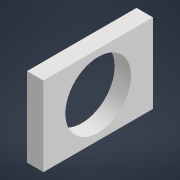
# Autodesk Inventor part: Part1
Saved by Autodesk Inventor 2022 (Build 260153000, 153)
## iProperties
Created: 2021-11-03
Part Number: Part1
Material: Generic
Document SubType Name: Modeling
Designer: 17185
Density: 1 g/cm^3
Appearance: Default
Author: 17185
Autodesk Inventor part; units mm, degrees
ref_plane "YZ Plane" through (0, 0, 0) normal (1, 0, 0) x (0, 1, 0)
ref_plane "XZ Plane" through (0, 0, 0) normal (0, 1, 0) x (-1, 0, 0)
ref_plane "XY Plane" through (0, 0, 0) normal (0, 0, 1) x (1, 0, 0)
sketch "Sketch1" plane through (0, 0, 0) normal (1, 0, 0) x (0, 1, 0)
  line L0 (46.0375, 63.5) -> (-46.0375, 63.5)
  line L1 (-46.0375, 63.5) -> (-46.0375, -63.5)
  line L2 (-46.0375, -63.5) -> (46.0375, -63.5)
  line L3 (46.0375, -63.5) -> (46.0375, 63.5)
  line L4 (46.0375, 63.5) -> (-46.0375, -63.5) construction
  line L5 (-46.0375, 63.5) -> (46.0375, -63.5) construction
  circle A0 centre (0, 0) radius 38.1
  dimension "d0" = 92.075
  dimension "d1" = 127
  dimension "d4" = 76.2
  constraints: 12 end point, 2 midpoint, 2 parallel, 1 centre point, 1 coincident, 1 horizontal, 1 perpendicular
  measures "d0" distance of L1.end L2.end
  measures "d1" distance of L0.end L1.end
  measures "d4" diameter of A0
extrude "Extrusion1" add sketch "Sketch1" along normal blind 19.05
body "Solid1"
